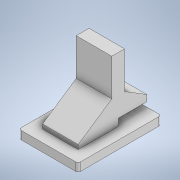
# Autodesk Inventor part: stopper
Saved by Autodesk Inventor 2021.1 (Build 251245010, 245A)
## iProperties
Created: 2021-08-22
Part Number: stopper
Material: Типовые
Document SubType Name: Modeling
Designer: User
Density: 1 g/cm^3
Appearance: По умолчанию
Author: User
Autodesk Inventor part; units mm, degrees
ref_plane "YZ Plane" through (0, 0, 0) normal (1, 0, 0) x (0, 1, 0)
ref_plane "XZ Plane" through (0, 0, 0) normal (0, 1, 0) x (-1, 0, 0)
ref_plane "XY Plane" through (0, 0, 0) normal (0, 0, 1) x (1, 0, 0)
sketch "Эскиз1" plane through (0, 0, 0) normal (0, 1, 0) x (-1, 0, 0)
  line L0 (-7.5, 14.5) -> (7.5, 14.5)
  line L1 (7.5, 14.5) -> (7.5, -14.5)
  line L2 (7.5, -14.5) -> (-7.5, -14.5)
  line L3 (-7.5, -14.5) -> (-7.5, 14.5)
  line L4 (-7.5, 14.5) -> (7.5, -14.5) construction
  line L5 (7.5, 14.5) -> (-7.5, -14.5) construction
  point P0 (0, 0)
  dimension "d0" = 15
  dimension "d1" = 29
  constraints: 12 end point, 2 midpoint, 2 parallel, 1 horizontal, 1 perpendicular
  measures "d0" distance of L1.end L2.end
  measures "d1" distance of L0.end L1.end
extrude "Выдавливание1" add sketch "Эскиз1" along normal blind 27
sketch "Эскиз2" plane through (0, 0, 0) normal (0, -1, 0) x (1, 0, 0)
  line L0 (12.5, 19.5) -> (-12.5, 19.5)
  line L1 (-12.5, 19.5) -> (-12.5, -15.5)
  line L2 (-12.5, -15.5) -> (12.5, -15.5)
  line L3 (12.5, -15.5) -> (12.5, 19.5)
  line L4 (7.5, 14.5) -> (7.5, -14.5) projected
  line L5 (-7.5, 14.5) -> (7.5, 14.5) projected
  point P0 (0, 0)
  dimension "d4" = 25
  dimension "d5" = 35
  dimension "d6" = 5
  dimension "d7" = 5
  constraints: 8 end point, 2 parallel, 1 horizontal, 1 perpendicular
  measures "d4" distance of L2.end L1.end
  measures "d5" distance of L1.end L0.end
  measures "d6" distance between parallel lines of L3 L4
  measures "d7" distance between parallel lines of L0 L5
extrude "Выдавливание2" add sketch "Эскиз2" along normal blind 3.5
fillet "Сопряжение1" radius 1 1 edges at (-12.5, -1.75, 19.5)
fillet "Сопряжение2" radius 1 2 edges at (12.5, -1.75, 19.5) (12.5, -1.75, -15.5)
fillet "Сопряжение3" radius 1 1 edges at (-12.5, -1.75, -15.5)
sketch "Эскиз3" plane through (7.5, 27, 14.5) normal (1, 0, 0) x (0, 0, -1)
  line L0 (14.2, 0) -> (14.2, -15.6)
  line L1 (0, -27) -> (0, 0) projected
  line L2 (0, 0) -> (29, 0) projected
  line L3 (29, -27) -> (-4, -27) projected
  line L4 (0, -25.2) -> (14.2, -15.6)
  line L5 (-4, -27) -> (29, -27) projected
  line L6 (17, -27) -> (17, -24)
  line L7 (17, -24) -> (29, -24)
  line L8 (29, -27) -> (29, 0) projected
  line L9 (29, 0) -> (0, 0) projected
  line L10 (19.6, 0) -> (19.6, -15.6)
  line L11 (19.6, -15.6) -> (29, -21.4)
  point P0 (14.5, -27)
  dimension "d13" = 14.2
  dimension "d16" = 17
  dimension "d17" = 3
  dimension "d18" = 9.4
  constraints: 12 end point, 6 point on line, 2 perpendicular, 1 horizontal, 1 vertical
  measures "d13" distance between parallel lines of L1 L0
  measures "d16" distance between parallel lines of L1 L6
  measures "d17" distance between parallel lines of L3 L7
  measures "d18" distance between parallel lines of L10 L8
extrude "Выдавливание3" cut sketch "Эскиз3" against normal blind 23 contours L0 L4 L1 L2 | L2 L8 L11 L10 | L6 L7 L8 L3
